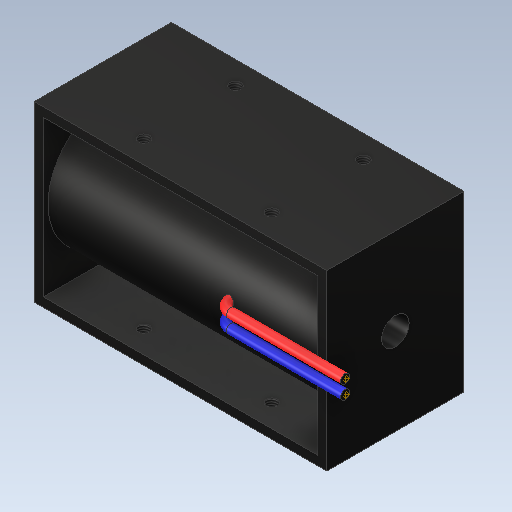
# Autodesk Inventor part: Korper
Saved by Autodesk Inventor 2020 (Build 240168000, 168)
## iProperties
Created: 2020-03-06
Part Number: Korper
Material: Generisch
Document SubType Name: Modeling
Designer: kaebi
Density: 1 g/cm^3
Appearance: Glänzend - Schwarz
Author: kaebi
Autodesk Inventor part; units mm, degrees
ref_plane "YZ Plane" through (0, 0, 0) normal (1, 0, 0) x (0, 1, 0)
ref_plane "XZ Plane" through (0, 0, 0) normal (0, 1, 0) x (-1, 0, 0)
ref_plane "XY Plane" through (0, 0, 0) normal (0, 0, 1) x (1, 0, 0)
sketch "Skizze1" plane through (0, 0, 0) normal (0, 0, 1) x (1, 0, 0)
  line L0 (-30, -17) -> (30, -17)
  line L1 (30, -17) -> (30, 17)
  line L2 (30, 17) -> (-30, 17)
  line L3 (-30, 17) -> (-30, -17)
  line L4 (-30, -17) -> (30, 17) construction
  line L5 (30, -17) -> (-30, 17) construction
  line L6 (-32, -19) -> (32, -19)
  line L7 (32, -19) -> (32, 19)
  line L8 (32, 19) -> (-32, 19)
  line L9 (-32, 19) -> (-32, -19)
  line L10 (-32, -19) -> (32, 19) construction
  line L11 (32, -19) -> (-32, 19) construction
  point P0 (0, 0)
  dimension "d0" = 38
  dimension "d1" = 64
  dimension "d2" = 2
  dimension "d3" = 2
  constraints: 24 end point, 4 midpoint, 4 parallel, 2 horizontal, 2 perpendicular
  measures "d0" distance of L6.end L7.end
  measures "d1" distance of L7.end L8.end
  measures "d2" distance between parallel lines of L8 L2
  measures "d3" distance between parallel lines of L7 L1
extrude "Extrusion1" add sketch "Skizze1" along normal mid plane 30
sketch "Skizze2" plane through (-30, -17, -15) normal (1, 0, 0) x (0, 0, -1)
  circle A0 centre (-15, 17) radius 14
  dimension "d6" = 28
  constraints: 1 centre point, 1 coincident
  measures "d6" diameter of A0
extrude "Extrusion2" add sketch "Skizze2" along normal up to next
sketch "Skizze3" plane through (32, -19, 15) normal (1, 0, 0) x (0, 0, -1)
  circle A0 centre (15, 19) radius 3
  dimension "d9" = 6
  constraints: 1 centre point, 1 coincident
  measures "d9" diameter of A0
extrude "Extrusion3" cut sketch "Skizze3" against normal through all
sketch "Skizze4" plane through (-32, -19, 15) normal (-1, 0, 0) x (0, 0, 1)
  circle A0 centre (-15, 19) radius 8
  dimension "d12" = 16
  constraints: 1 centre point, 1 coincident
  measures "d12" diameter of A0
extrude "Extrusion4" cut sketch "Skizze4" against normal blind 30
sketch "Skizze5" plane through (-32, 19, 15) normal (0, 1, 0) x (1, 0, 0)
  line L0 (19, 5) -> (47, 5)
  line L1 (47, 5) -> (47, 25)
  line L2 (47, 25) -> (19, 25)
  line L3 (19, 25) -> (19, 5)
  line L4 (19, 5) -> (47, 25) construction
  line L5 (47, 5) -> (19, 25) construction
  line L6 (64, 30) -> (64, 0) projected
  point P0 (32, 15)
  point P1 (33, 15)
  point P2 (33, 15)
  dimension "d15" = 28
  dimension "d16" = 20
  dimension "d17" = 17
  constraints: 12 end point, 4 coincident, 3 midpoint, 2 parallel, 1 horizontal, 1 horizontal alignment, 1 perpendicular
  measures "d15" distance of L1.end L2.end
  measures "d16" distance of L0.end L1.end
  measures "d17" distance between parallel lines of L6 L1
hole "Bohrung1" at (-13, 19, -10) at (15, 19, -10) at (15, 19, 10) at (-13, 19, 10) direction (0, -1, 0) diameter 2.459 depth 2 thread size "M3x0.5" class "6H" standard "ISO Metric profile"
sketch "Skizze6" plane through (-32, -19, 15) normal (0, -1, 0) x (1, 0, 0)
  circle A0 centre (47, -5) radius 1.2295 projected
  circle A1 centre (19, -25) radius 1.2295 projected
  circle A2 centre (47, -25) radius 1.2295 projected
  circle A3 centre (19, -5) radius 1.2295 projected
  line L0 (2, -30) -> (2, 0) projected
  line L1 (62, -30) -> (2, -30) projected
  line L2 (62, -30) -> (62, 0) projected
  line L3 (2, 0) -> (62, 0) projected
  point P0 (32, -15)
  constraints: 4 coincident
hole "Bohrung2" at (-13, -19, 10) at (-13, -19, -10) at (15, -19, -10) at (15, -19, 10) direction (0, 1, 0) diameter 2.459 depth 2 thread size "M3x0.5" class "6H" standard "ISO Metric profile"
sketch "Skizze7" plane through (32, -19, 15) normal (1, 0, 0) x (0, 0, -1)
  circle A0 centre (-1, 20.5) radius 1
  circle A1 centre (-1, 17.5) radius 1
  line L0 (0, 0) -> (0, 38) projected
  line L1 (36.4, 19) -> (-8.4, 19) projected
  point P0 (15, 19)
  dimension "d32" = 2
  dimension "d34" = 3
  dimension "d35" = 1
  constraints: 2 centre point, 1 equal radius, 1 symmetric about line, 1 vertical alignment
  measures "d32" diameter of A0
  measures "d34" distance of A0.centre A1.centre
  measures "d35" distance from line of L0 A0.centre
extrude "Extrusion5" add sketch "Skizze7" along normal blind 5 and the other way blind 20
sketch "Skizze8" plane through (12, 1.5, 16) normal (-1, 0, 0) x (0, 0, 1)
  circle A0 centre (0, -3) radius 1 projected
  circle A1 centre (0, 0) radius 1 projected
  circle A2 centre (0, -3) radius 1
  circle A3 centre (0, 0) radius 1
  circle A4 centre (-16, -1.5) radius 14 projected
  line L0 (-2.5175, -5.2711) -> (-2.5175, 7.0646)
  point P0 (-16, -1.5)
  constraints: 2 centre point, 2 coincident, 2 end point, 1 concentric, 1 vertical, 2 other
revolve "Umdrehung1" add sketch "Skizze8" angle 90 about axis through (12, -3.7711, 13.4825) along (0, -1, 0) contours A0 | A1
sketch "Skizze9" plane through (37, 1.5, 16) normal (1, 0, 0) x (0, 0, -1)
  circle A0 centre (0, 0) radius 1 projected
sketch "Skizze10" plane through (37, -1.5, 16) normal (1, 0, 0) x (0, 0, -1)
  circle A0 centre (0, 0) radius 1 projected
